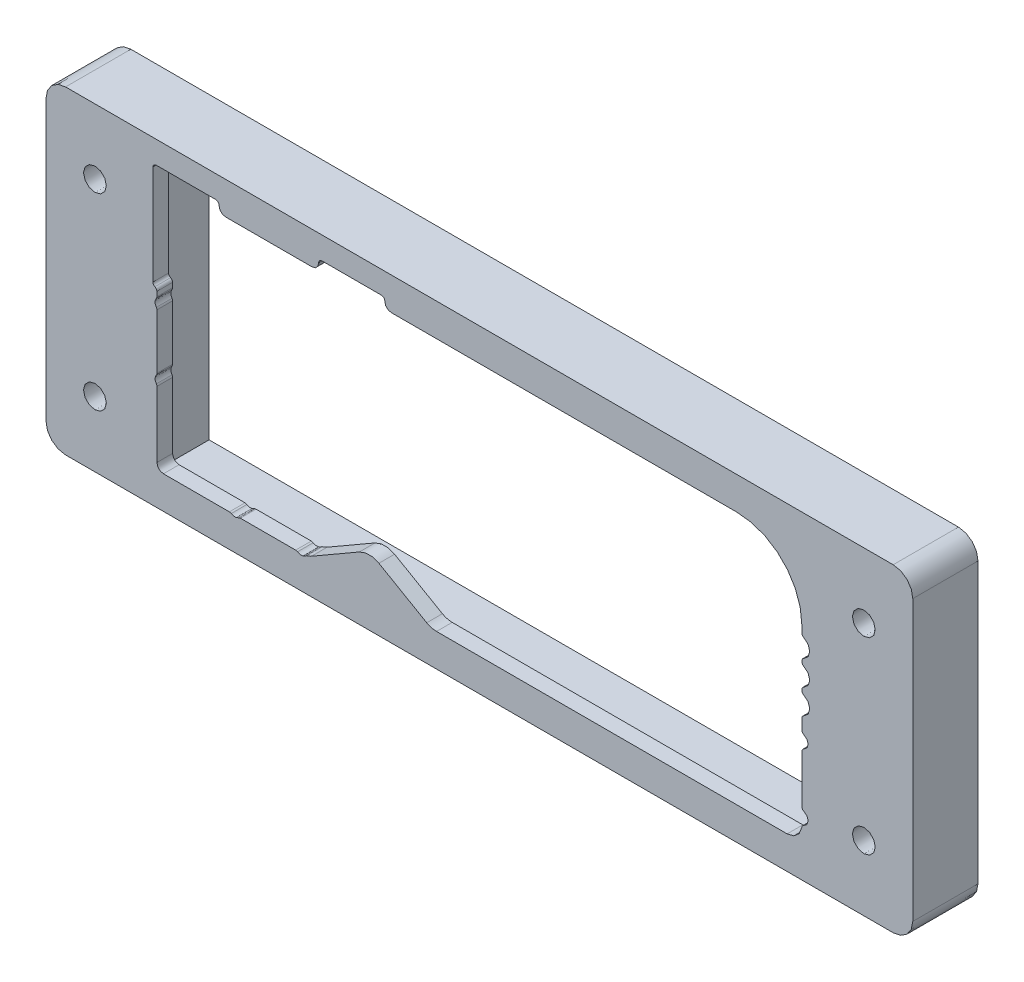
# Autodesk Inventor part: LCD-Halterung
Saved by Autodesk Inventor 2017.3 (Build 213256000, 256)
## iProperties
Part Number: LCD-Halterung
Material: Generisch
Document SubType Name: Modeling
Designer: Nils
Density: 1 g/cm^3
Appearance: Vorgabe
Author: Nils
Autodesk Inventor part; units mm, degrees
ref_plane "YZ Plane" through (0, 0, 0) normal (1, 0, 0) x (0, 1, 0)
ref_plane "XZ Plane" through (0, 0, 0) normal (0, 1, 0) x (-1, 0, 0)
ref_plane "XY Plane" through (0, 0, 0) normal (0, 0, 1) x (1, 0, 0)
sketch "Skizze1" plane through (0, 0, 0) normal (0, 0, 1) x (1, 0, 0)
  circle A0 centre (-4.2343, -14.8275) radius 0.85 projected
  circle A1 centre (35.7657, -14.8275) radius 0.85 projected
  circle A2 centre (-10.8343, -16.0775) radius 0.75 projected
  circle A3 centre (42.3657, -16.0775) radius 0.75 projected
  circle A4 centre (46.4957, 0.0825) radius 0.66 projected
  circle A5 centre (46.4957, 3.8925) radius 0.66 projected
  circle A6 centre (46.4957, 7.7025) radius 0.66 projected
  circle A7 centre (-44.7343, -15.1575) radius 0.5 projected
  circle A8 centre (-29.9543, -17.4975) radius 0.455 projected
  circle A9 centre (-40.1143, -17.4975) radius 0.455 projected
  circle A10 centre (-29.9543, -9.8775) radius 0.455 projected
  circle A11 centre (-40.1143, -9.8775) radius 0.455 projected
  circle A12 centre (-29.9543, 7.5025) radius 0.455 projected
  circle A13 centre (-40.1143, 7.5025) radius 0.455 projected
  circle A14 centre (-29.9543, 15.1225) radius 0.455 projected
  circle A15 centre (-40.1143, 15.1225) radius 0.455 projected
  circle A16 centre (-51.3443, -6.2675) radius 0.455 projected
  circle A17 centre (-51.3443, 3.8925) radius 0.455 projected
  circle A18 centre (-43.7243, -6.2675) radius 0.455 projected
  circle A19 centre (-43.7243, 3.8925) radius 0.455 projected
  circle A20 centre (-26.3443, -6.2675) radius 0.455 projected
  circle A21 centre (-26.3443, 3.8925) radius 0.455 projected
  circle A22 centre (-18.7243, -6.2675) radius 0.455 projected
  circle A23 centre (-18.7243, 3.8925) radius 0.455 projected
  circle A24 centre (-38.8443, -6.2675) radius 0.455 projected
  circle A25 centre (-38.8443, 3.8925) radius 0.455 projected
  circle A26 centre (-31.2243, -6.2675) radius 0.455 projected
  circle A27 centre (-31.2243, 3.8925) radius 0.455 projected
  circle A28 centre (-21.0643, 11.5125) radius 0.455 projected
  circle A29 centre (-23.6043, 11.5125) radius 0.455 projected
  circle A30 centre (-21.0643, 14.0525) radius 0.455 projected
  circle A31 centre (-23.6043, 14.0525) radius 0.455 projected
  circle A32 centre (-21.0643, 16.5925) radius 0.455 projected
  circle A33 centre (-23.6043, 16.5925) radius 0.455 projected
  circle A34 centre (-46.4643, 11.5125) radius 0.455 projected
  circle A35 centre (-49.0043, 11.5125) radius 0.455 projected
  circle A36 centre (-46.4643, 14.0525) radius 0.455 projected
  circle A37 centre (-49.0043, 14.0525) radius 0.455 projected
  circle A38 centre (-46.4643, 16.5925) radius 0.455 projected
  circle A39 centre (-49.0043, 16.5925) radius 0.455 projected
  circle A40 centre (46.7557, -14.9075) radius 0.405 projected
  circle A41 centre (46.7557, -4.7475) radius 0.405 projected
  circle A42 centre (-47.7343, -10.3575) radius 0.4 projected
  circle A43 centre (-50.7343, -15.1575) radius 0.4 projected
  circle A44 centre (16.3957, -17.6275) radius 0.3 projected
  circle A45 centre (17.6757, -17.6275) radius 0.3 projected
  circle A46 centre (15.1257, -17.6275) radius 0.3 projected
  circle A47 centre (25.2857, -17.6275) radius 0.3 projected
  circle A48 centre (26.5657, -17.6275) radius 0.3 projected
  circle A49 centre (27.8357, -17.6275) radius 0.3 projected
  circle A50 centre (29.0957, -17.6275) radius 0.3 projected
  circle A51 centre (30.3657, -17.6275) radius 0.3 projected
  circle A52 centre (32.9057, -17.6275) radius 0.3 projected
  circle A53 centre (13.8557, -17.6275) radius 0.3 projected
  circle A54 centre (12.5957, -17.6275) radius 0.3 projected
  circle A55 centre (11.3157, -17.6275) radius 0.3 projected
  circle A56 centre (10.0457, -17.6275) radius 0.3 projected
  circle A57 centre (8.7757, -17.6275) radius 0.3 projected
  circle A58 centre (7.5057, -17.6275) radius 0.3 projected
  circle A59 centre (6.2457, -17.6275) radius 0.3 projected
  circle A60 centre (4.9657, -17.6275) radius 0.3 projected
  circle A61 centre (-1.3843, -17.6275) radius 0.3 projected
  circle A62 centre (18.9357, -17.6275) radius 0.3 projected
  circle A63 centre (24.0157, -17.6275) radius 0.3 projected
  circle A64 centre (22.7457, -17.6275) radius 0.3 projected
  circle A65 centre (20.2057, -17.6275) radius 0.3 projected
  circle A66 centre (21.4757, -17.6275) radius 0.3 projected
  circle A67 centre (31.6357, -17.6275) radius 0.3 projected
  circle A68 centre (1.1557, -17.6275) radius 0.3 projected
  circle A69 centre (2.4257, -17.6275) radius 0.3 projected
  circle A70 centre (-0.1143, -17.6275) radius 0.3 projected
  circle A71 centre (3.7057, -17.6275) radius 0.3 projected
  circle A72 centre (26.1797, 7.9565) radius 0.175 projected
  circle A73 centre (24.6557, 3.0035) radius 0.175 projected
  circle A74 centre (16.4007, -1.3145) radius 0.175 projected
  circle A75 centre (16.4007, -0.1715) radius 0.175 projected
  circle A76 centre (16.4007, 1.8605) radius 0.175 projected
  circle A77 centre (-9.8883, 7.0675) radius 0.175 projected
  circle A78 centre (17.5437, 8.3375) radius 0.175 projected
  circle A79 centre (17.5437, 9.3535) radius 0.175 projected
  circle A80 centre (17.5437, 10.3695) radius 0.175 projected
  circle A81 centre (26.1797, 8.7185) radius 0.175 projected
  circle A82 centre (-0.1093, -15.1575) radius 0.175 projected
  circle A83 centre (25.4177, -2.3305) radius 0.175 projected
  circle A84 centre (25.4177, 0.0825) radius 0.175 projected
  circle A85 centre (21.9887, 13.4175) radius 0.175 projected
  circle A86 centre (26.1797, 0.0825) radius 0.175 projected
  circle A87 centre (22.7507, 14.0525) radius 0.175 projected
  circle A88 centre (2.0497, -8.2995) radius 0.175 projected
  circle A89 centre (31.5216, 5.0434) radius 0.175 projected
  circle A90 centre (9.0347, 14.1795) radius 0.175 projected
  circle A91 centre (0.7797, 14.4335) radius 0.175 projected
  circle A92 centre (-2.1413, 14.3065) radius 0.175 projected
  circle A93 centre (14.4957, 11.5125) radius 0.175 projected
  circle A94 centre (-6.7133, -8.2995) radius 0.175 projected
  circle A95 centre (4.7167, -5.6325) radius 0.175 projected
  circle A96 centre (4.7167, 4.5275) radius 0.175 projected
  circle A97 centre (27.8307, -6.6485) radius 0.175 projected
  circle A98 centre (16.6547, -10.2045) radius 0.175 projected
  circle A99 centre (1.1607, -14.3955) radius 0.175 projected
  circle A100 centre (40.7847, 8.2105) radius 0.175 projected
  circle A101 centre (18.5597, 16.0845) radius 0.175 projected
  circle A102 centre (4.3357, 13.7985) radius 0.175 projected
  circle A103 centre (30.6247, 6.9405) radius 0.175 projected
  circle A104 centre (28.9737, 5.2895) radius 0.175 projected
  circle A105 centre (10.0507, -11.2205) radius 0.175 projected
  circle A106 centre (20.9727, 11.7665) radius 0.175 projected
  line L0 (48.7857, -20.2375) -> (-54.0643, -20.2375) projected
  line L1 (48.7857, 22.6125) -> (48.7857, -20.2375) projected
  line L2 (-54.0643, 22.6125) -> (48.7857, 22.6125) projected
  line L3 (-54.0643, -20.2375) -> (-54.0643, 22.6125) projected
  line L4 (60.7857, -23.2375) -> (-66.0643, -23.2375)
  line L5 (-69.0643, -20.2375) -> (-69.0643, 22.6125)
  line L6 (-66.0643, 25.6125) -> (60.7857, 25.6125)
  line L7 (63.7857, 22.6125) -> (63.7857, -20.2375)
  arc A107 (60.7857, -23.2375) -> (63.7857, -20.2375) centre (60.7857, -20.2375) ccw
  arc A108 (63.7857, 22.6125) -> (60.7857, 25.6125) centre (60.7857, 22.6125) ccw
  arc A109 (-66.0643, 25.6125) -> (-69.0643, 22.6125) centre (-66.0643, 22.6125) ccw
  arc A110 (-69.0643, -20.2375) -> (-66.0643, -23.2375) centre (-66.0643, -20.2375) ccw
  point P0 (0, 0)
  dimension "d0" = 3
  dimension "d1" = 3
  dimension "d2" = 15
  dimension "d3" = 15
  dimension "d4" = 3
  constraints: 8 end point, 8 point on circle, 8 tangent, 4 centre point, 3 equal radius, 2 parallel, 1 horizontal, 1 perpendicular
  measures "d0" distance between parallel lines of L4 L0
  measures "d1" distance between parallel lines of L6 L2
  measures "d2" distance between parallel lines of L1 L7
  measures "d3" distance between parallel lines of L5 L3
  measures "d4" radius of A107
extrude "Extrusion1" add sketch "Skizze1" along normal blind 10 contours L4 A110 L5 A109 L6 A108 L7 A107
ref_plane "Arbeitsebene1" through (-2.6393, 1.1875, 7.6) normal (0, 0, 1) x (1, 0, 0)
sketch "Skizze2" plane through (-2.6393, 1.1875, 7.6) normal (0, 0, 1) x (1, 0, 0)
  line L0 (-51.425, -21.425) -> (-51.425, 21.425) projected
  line L1 (-51.425, 21.425) -> (51.425, 21.425) projected
  line L2 (51.425, 21.425) -> (51.425, -21.425) projected
  line L3 (51.425, -21.425) -> (-51.425, -21.425) projected
  line L4 (-63.425, -24.425) -> (63.425, -24.425) projected
  arc A0 (63.425, -24.425) -> (66.425, -21.425) centre (63.425, -21.425) ccw projected
  line L5 (66.425, -21.425) -> (66.425, 21.425) projected
  arc A1 (66.425, 21.425) -> (63.425, 24.425) centre (63.425, 21.425) ccw projected
  line L6 (63.425, 24.425) -> (-63.425, 24.425) projected
  arc A2 (-63.425, 24.425) -> (-66.425, 21.425) centre (-63.425, 21.425) ccw projected
  line L7 (-66.425, 21.425) -> (-66.425, -21.425) projected
  arc A3 (-66.425, -21.425) -> (-63.425, -24.425) centre (-63.425, -21.425) ccw projected
  line L8 (-8.0686, -19.0231) -> (-15.3987, -14.791)
  line L9 (-18.3987, -14.791) -> (-25.7288, -19.0231)
  line L10 (47.175, -19.425) -> (-6.5686, -19.425)
  arc A4 (-15.3987, -14.791) -> (-18.3987, -14.791) centre (-16.8987, -17.3891) ccw
  arc A5 (-26.4463, -19.3211) -> (-25.7288, -19.0231) centre (-27.2288, -16.425) ccw
  arc A6 (-8.0686, -19.0231) -> (-6.5686, -19.425) centre (-6.5686, -16.425) ccw
  arc A7 (-49.425, -18.425) -> (-48.425, -19.425) centre (-48.425, -18.425) ccw
  arc A8 (49.425, 9.425) -> (39.425, 19.425) centre (39.425, 9.425) ccw
  arc A9 (47.175, -19.425) -> (49.4027, -17.4913) centre (47.175, -17.175) ccw
  circle A10 centre (-1.595, -16.015) radius 0.85 construction
  circle A11 centre (38.405, -16.015) radius 0.85 construction
  circle A12 centre (-8.195, -17.265) radius 0.75 construction
  circle A13 centre (45.005, -17.265) radius 0.75 construction
  circle A14 centre (49.135, -1.105) radius 0.66 construction
  circle A15 centre (49.135, 2.705) radius 0.66 construction
  circle A16 centre (49.135, 6.515) radius 0.66 construction
  circle A17 centre (-42.095, -16.345) radius 0.5 construction
  circle A18 centre (-27.315, -18.685) radius 0.455 construction
  circle A19 centre (-37.475, -18.685) radius 0.455 construction
  circle A20 centre (-27.315, -11.065) radius 0.455 construction
  circle A21 centre (-37.475, -11.065) radius 0.455 construction
  circle A22 centre (-27.315, 6.315) radius 0.455 construction
  circle A23 centre (-37.475, 6.315) radius 0.455 construction
  circle A24 centre (-27.315, 13.935) radius 0.455 construction
  circle A25 centre (-37.475, 13.935) radius 0.455 construction
  circle A26 centre (-48.705, -7.455) radius 0.455 construction
  circle A27 centre (-48.705, 2.705) radius 0.455 construction
  circle A28 centre (-41.085, -7.455) radius 0.455 construction
  circle A29 centre (-41.085, 2.705) radius 0.455 construction
  circle A30 centre (-23.705, -7.455) radius 0.455 construction
  circle A31 centre (-23.705, 2.705) radius 0.455 construction
  circle A32 centre (-16.085, -7.455) radius 0.455 construction
  circle A33 centre (-16.085, 2.705) radius 0.455 construction
  circle A34 centre (-36.205, -7.455) radius 0.455 construction
  circle A35 centre (-36.205, 2.705) radius 0.455 construction
  circle A36 centre (-28.585, -7.455) radius 0.455 construction
  circle A37 centre (-28.585, 2.705) radius 0.455 construction
  circle A38 centre (-18.425, 10.325) radius 0.455 construction
  circle A39 centre (-20.965, 10.325) radius 0.455 construction
  circle A40 centre (-18.425, 12.865) radius 0.455 construction
  circle A41 centre (-20.965, 12.865) radius 0.455 construction
  circle A42 centre (-18.425, 15.405) radius 0.455 construction
  circle A43 centre (-20.965, 15.405) radius 0.455 construction
  circle A44 centre (-43.825, 10.325) radius 0.455 construction
  circle A45 centre (-46.365, 10.325) radius 0.455 construction
  circle A46 centre (-43.825, 12.865) radius 0.455 construction
  circle A47 centre (-46.365, 12.865) radius 0.455 construction
  circle A48 centre (-43.825, 15.405) radius 0.455 construction
  circle A49 centre (-46.365, 15.405) radius 0.455 construction
  circle A50 centre (49.395, -16.095) radius 0.405 construction
  circle A51 centre (49.395, -5.935) radius 0.405 construction
  circle A52 centre (-45.095, -11.545) radius 0.4 construction
  circle A53 centre (-48.095, -16.345) radius 0.4 construction
  circle A54 centre (19.035, -18.815) radius 0.3 construction
  circle A55 centre (20.315, -18.815) radius 0.3 construction
  circle A56 centre (17.765, -18.815) radius 0.3 construction
  circle A57 centre (27.925, -18.815) radius 0.3 construction
  circle A58 centre (29.205, -18.815) radius 0.3 construction
  circle A59 centre (30.475, -18.815) radius 0.3 construction
  circle A60 centre (31.735, -18.815) radius 0.3 construction
  circle A61 centre (33.005, -18.815) radius 0.3 construction
  circle A62 centre (35.545, -18.815) radius 0.3 construction
  circle A63 centre (16.495, -18.815) radius 0.3 construction
  circle A64 centre (15.235, -18.815) radius 0.3 construction
  circle A65 centre (13.955, -18.815) radius 0.3 construction
  circle A66 centre (12.685, -18.815) radius 0.3 construction
  circle A67 centre (11.415, -18.815) radius 0.3 construction
  circle A68 centre (10.145, -18.815) radius 0.3 construction
  circle A69 centre (8.885, -18.815) radius 0.3 construction
  circle A70 centre (7.605, -18.815) radius 0.3 construction
  circle A71 centre (1.255, -18.815) radius 0.3 construction
  circle A72 centre (21.575, -18.815) radius 0.3 construction
  circle A73 centre (26.655, -18.815) radius 0.3 construction
  circle A74 centre (25.385, -18.815) radius 0.3 construction
  circle A75 centre (22.845, -18.815) radius 0.3 construction
  circle A76 centre (24.115, -18.815) radius 0.3 construction
  circle A77 centre (34.275, -18.815) radius 0.3 construction
  circle A78 centre (3.795, -18.815) radius 0.3 construction
  circle A79 centre (5.065, -18.815) radius 0.3 construction
  circle A80 centre (2.525, -18.815) radius 0.3 construction
  circle A81 centre (6.345, -18.815) radius 0.3 construction
  circle A82 centre (28.819, 6.769) radius 0.175 construction
  circle A83 centre (27.295, 1.816) radius 0.175 construction
  circle A84 centre (19.04, -2.502) radius 0.175 construction
  circle A85 centre (19.04, -1.359) radius 0.175 construction
  circle A86 centre (19.04, 0.673) radius 0.175 construction
  circle A87 centre (-7.249, 5.88) radius 0.175 construction
  circle A88 centre (20.183, 7.15) radius 0.175 construction
  circle A89 centre (20.183, 8.166) radius 0.175 construction
  circle A90 centre (20.183, 9.182) radius 0.175 construction
  circle A91 centre (28.819, 7.531) radius 0.175 construction
  circle A92 centre (2.53, -16.345) radius 0.175 construction
  circle A93 centre (28.057, -3.518) radius 0.175 construction
  circle A94 centre (28.057, -1.105) radius 0.175 construction
  circle A95 centre (24.628, 12.23) radius 0.175 construction
  circle A96 centre (28.819, -1.105) radius 0.175 construction
  circle A97 centre (25.39, 12.865) radius 0.175 construction
  circle A98 centre (4.689, -9.487) radius 0.175 construction
  circle A99 centre (34.1609, 3.8559) radius 0.175 construction
  circle A100 centre (11.674, 12.992) radius 0.175 construction
  circle A101 centre (3.419, 13.246) radius 0.175 construction
  circle A102 centre (0.498, 13.119) radius 0.175 construction
  circle A103 centre (17.135, 10.325) radius 0.175 construction
  circle A104 centre (-4.074, -9.487) radius 0.175 construction
  circle A105 centre (7.356, -6.82) radius 0.175 construction
  circle A106 centre (7.356, 3.34) radius 0.175 construction
  circle A107 centre (30.47, -7.836) radius 0.175 construction
  circle A108 centre (19.294, -11.392) radius 0.175 construction
  circle A109 centre (3.8, -15.583) radius 0.175 construction
  circle A110 centre (43.424, 7.023) radius 0.175 construction
  circle A111 centre (21.199, 14.897) radius 0.175 construction
  circle A112 centre (6.975, 12.611) radius 0.175 construction
  circle A113 centre (33.264, 5.753) radius 0.175 construction
  circle A114 centre (31.613, 4.102) radius 0.175 construction
  circle A115 centre (12.69, -12.408) radius 0.175 construction
  circle A116 centre (23.612, 10.579) radius 0.175 construction
  line L11 (51.425, -21.425) -> (-51.425, -21.425) construction
  line L12 (51.425, 21.425) -> (51.425, -21.425) construction
  line L13 (-51.425, 21.425) -> (51.425, 21.425) construction
  line L14 (-51.425, -21.425) -> (-51.425, 21.425) construction
  line L15 (-40.396, 5.245) -> (-40.396, 20.485) construction
  line L16 (-40.396, 20.485) -> (-49.54, 20.485) construction
  line L17 (-49.54, 20.485) -> (-49.54, 5.245) construction
  line L18 (-49.54, 5.245) -> (-40.396, 5.245) construction
  line L19 (-14.996, 5.245) -> (-14.996, 20.485) construction
  line L20 (-14.996, 20.485) -> (-24.14, 20.485) construction
  line L21 (-24.14, 20.485) -> (-24.14, 5.245) construction
  line L22 (-24.14, 5.245) -> (-14.996, 5.245) construction
  line L23 (-27.995, -20.075) -> (-27.395, -20.075) construction
  line L24 (-27.395, -20.075) -> (-27.395, -18.895) construction
  line L25 (-28.185, -20.305) -> (-28.3918, -20.305) construction
  line L26 (-28.7782, -20.305) -> (-28.3918, -20.305) construction
  line L27 (-28.7782, -20.305) -> (-28.985, -20.305) construction
  line L28 (-28.985, -20.075) -> (-30.725, -20.075) construction
  line L29 (-31.525, -20.075) -> (-30.725, -20.075) construction
  line L30 (-33.065, -20.075) -> (-34.525, -20.075) construction
  line L31 (-35.595, -20.075) -> (-34.595, -20.075) construction
  line L32 (-36.3982, -20.305) -> (-36.0118, -20.305) construction
  line L33 (-37.395, -20.075) -> (-36.795, -20.075) construction
  line L34 (-37.395, -18.895) -> (-37.395, -20.075) construction
  line L35 (-50.095, -6.195) -> (-50.095, -7.375) construction
  line L36 (-50.095, -6.195) -> (-50.095, -5.555) construction
  line L37 (-50.095, -4.175) -> (-50.095, -0.575) construction
  line L38 (-50.095, 2.625) -> (-50.095, 1.445) construction
  line L39 (-50.095, -7.375) -> (-49.495, -7.375) construction
  line L40 (-49.495, 2.625) -> (-50.095, 2.625) construction
  arc A117 (-27.8777, -19.5117) -> (-26.6489, -19.4309) centre (-27.315, -18.685) ccw
  arc A118 (-38.0377, -19.5117) -> (-36.9123, -19.5117) centre (-37.475, -18.685) ccw
  line L41 (-28.159, -19.425) -> (-36.631, -19.425)
  line L42 (-38.319, -19.425) -> (-48.425, -19.425)
  arc A119 (49.7333, -17.036) -> (49.7483, -15.1595) centre (49.395, -16.095) ccw
  arc A120 (49.7483, -6.8705) -> (49.7483, -4.9995) centre (49.395, -5.935) ccw
  arc A121 (49.7275, -2.483) -> (49.7275, 0.273) centre (49.135, -1.105) ccw
  arc A122 (49.7275, 1.327) -> (49.7275, 4.083) centre (49.135, 2.705) ccw
  arc A123 (49.7275, 5.137) -> (49.7275, 7.893) centre (49.135, 6.515) ccw
  line L43 (49.425, -7.3382) -> (49.425, -14.6918)
  line L44 (49.425, -2.9424) -> (49.425, -4.5318)
  line L45 (49.425, 0.8676) -> (49.425, 0.7324)
  line L46 (49.425, 9.425) -> (49.425, 8.3524)
  line L47 (49.425, 4.6776) -> (49.425, 4.5424)
  line L48 (-24.64, 20.425) -> (-24.64, 20.485)
  line L49 (-24.14, 20.985) -> (-14.996, 20.985)
  line L50 (-14.496, 20.485) -> (-14.496, 20.425)
  line L51 (-50.04, 5.2116) -> (-50.04, 20.485)
  line L52 (-49.54, 20.985) -> (-40.396, 20.985)
  line L53 (-39.896, 20.485) -> (-39.896, 20.425)
  line L54 (-38.896, 19.425) -> (-25.64, 19.425)
  line L55 (-13.496, 19.425) -> (39.425, 19.425)
  arc A124 (-49.5183, -6.8732) -> (-49.5183, -8.0368) centre (-48.705, -7.455) ccw
  arc A125 (-49.5183, 3.2868) -> (-49.5183, 2.1232) centre (-48.705, 2.705) ccw
  line L56 (-49.425, 3.5777) -> (-49.425, 4.2884)
  line L57 (-49.425, -18.425) -> (-49.425, -8.3277)
  line L58 (-49.425, -6.5823) -> (-49.425, 1.8323)
  arc A126 (-14.496, 20.425) -> (-13.496, 19.425) centre (-13.496, 20.425) ccw
  arc A127 (-25.64, 19.425) -> (-24.64, 20.425) centre (-25.64, 20.425) ccw
  arc A128 (-39.896, 20.425) -> (-38.896, 19.425) centre (-38.896, 20.425) ccw
  arc A129 (-49.425, 4.2884) -> (-49.7326, 4.7502) centre (-49.9255, 4.2884) ccw
  arc A130 (49.425, 8.3524) -> (49.7275, 7.893) centre (49.925, 8.3524) ccw
  arc A131 (49.7275, 5.137) -> (49.425, 4.6776) centre (49.925, 4.6776) ccw
  arc A132 (49.425, 4.5424) -> (49.7275, 4.083) centre (49.925, 4.5424) ccw
  arc A133 (49.7275, 1.327) -> (49.425, 0.8676) centre (49.925, 0.8676) ccw
  arc A134 (49.425, 0.7324) -> (49.7275, 0.273) centre (49.925, 0.7324) ccw
  arc A135 (49.7275, -2.483) -> (49.425, -2.9424) centre (49.925, -2.9424) ccw
  arc A136 (49.425, -4.5318) -> (49.7483, -4.9995) centre (49.925, -4.5318) ccw
  arc A137 (49.7483, -6.8705) -> (49.425, -7.3382) centre (49.925, -7.3382) ccw
  arc A138 (49.425, -14.6918) -> (49.7483, -15.1595) centre (49.925, -14.6918) ccw
  arc A139 (49.7333, -17.036) -> (49.4027, -17.4913) centre (49.9024, -17.5066) ccw
  arc A140 (-39.896, 20.485) -> (-40.396, 20.985) centre (-40.396, 20.485) ccw
  arc A141 (-49.54, 20.985) -> (-50.04, 20.485) centre (-49.54, 20.485) ccw
  arc A142 (-24.14, 20.985) -> (-24.64, 20.485) centre (-24.14, 20.485) ccw
  arc A143 (-14.496, 20.485) -> (-14.996, 20.985) centre (-14.996, 20.485) ccw
  arc A144 (-50.04, 5.2116) -> (-49.7326, 4.7502) centre (-49.54, 5.2116) ccw
  arc A145 (-49.5183, 3.2868) -> (-49.425, 3.5777) centre (-49.925, 3.5777) ccw
  arc A146 (-49.425, 1.8323) -> (-49.5183, 2.1232) centre (-49.925, 1.8323) ccw
  arc A147 (-49.5183, -6.8732) -> (-49.425, -6.5823) centre (-49.925, -6.5823) ccw
  arc A148 (-49.425, -8.3277) -> (-49.5183, -8.0368) centre (-49.925, -8.3277) ccw
  arc A149 (-38.0377, -19.5117) -> (-38.319, -19.425) centre (-38.319, -19.925) ccw
  arc A150 (-36.631, -19.425) -> (-36.9123, -19.5117) centre (-36.631, -19.925) ccw
  arc A151 (-27.8777, -19.5117) -> (-28.159, -19.425) centre (-28.159, -19.925) ccw
  arc A152 (-26.4463, -19.3211) -> (-26.6489, -19.4309) centre (-26.3159, -19.8038) ccw
  point P0 (2.6393, -1.1875)
  point P1 (-49.425, -19.425)
  point P2 (-7.3724, -19.425)
  point P3 (-16.8987, -13.925)
  point P4 (-26.425, -19.425)
  point P5 (-49.425, 4.745)
  point P6 (-27.9876, -19.425)
  point P7 (-38.1476, -19.425)
  point P8 (-36.8024, -19.425)
  point P9 (49.425, -15.0955)
  point P10 (49.425, -17.0945)
  point P11 (49.425, -6.9345)
  point P12 (49.425, -4.9355)
  point P13 (49.425, -2.5767)
  point P14 (49.425, 0.3667)
  point P15 (49.425, 1.2333)
  point P16 (49.425, 4.1767)
  point P17 (49.425, 5.0433)
  point P18 (49.425, 7.9867)
  point P19 (-14.496, 19.425)
  point P20 (-24.64, 20.985)
  point P21 (-14.496, 20.985)
  point P22 (-50.04, 20.985)
  point P23 (-50.04, 4.745)
  point P24 (-39.896, 20.985)
  point P25 (-24.64, 19.425)
  point P26 (-39.896, 19.425)
  point P27 (-49.425, 2.011)
  point P28 (-49.425, 3.399)
  point P29 (-49.425, -8.149)
  point P30 (-49.425, -6.761)
  dimension "d11" = 120
  dimension "d13" = 23
  dimension "d14" = 2
  dimension "d16" = 5.5
  dimension "d17" = 3
  dimension "d18" = 3
  dimension "d19" = 1
  dimension "d20" = 2
  dimension "d21" = 2
  dimension "d22" = 2
  dimension "d23" = 2
  dimension "d24" = 3
  dimension "d25" = 3
  dimension "d26" = 3
  dimension "d27" = 0.5
  dimension "d28" = 0.5
  dimension "d29" = 0.5
  dimension "d30" = 0.5
  dimension "d31" = 0.5
  dimension "d33" = 2
  dimension "d34" = 2
  dimension "d37" = 2
  dimension "d38" = 2
  dimension "d39" = 10
  dimension "d40" = 2.25
  dimension "d52" = 1
  dimension "d54" = 0.5
  dimension "d55" = 0.5
  dimension "d56" = 0.5
  constraints: 101 point on circle, 77 tangent, 42 centre point, 42 end point, 38 point on line, 23 equal radius, 23 parallel, 9 coincident, 9 perpendicular, 3 horizontal, 1 equal length, 1 other
  measures "d11" angle of L9 L8
  measures "d13" distance of point (-49.425, -19.425) point (-26.425, -19.425)
  measures "d14" distance between parallel lines of L3 L10
  measures "d16" vertical distance of point (-7.372, -19.425) point (-16.899, -13.925)
  measures "d17" radius of A4
  measures "d18" radius of A6
  measures "d19" radius of A7
  measures "d20" diameter of A117
  measures "d21" diameter of A118
  measures "d22" diameter of A119
  measures "d23" diameter of A120
  measures "d24" diameter of A121
  measures "d25" diameter of A122
  measures "d26" diameter of A123
  measures "d27" distance between parallel lines of L20 L49
  measures "d28" distance between parallel lines of L19 L50
  measures "d29" distance between parallel lines of L48 L21
  measures "d30" distance between parallel lines of L15 L53
  measures "d31" distance between parallel lines of L51 L17
  measures "d33" diameter of A124
  measures "d34" diameter of A125
  measures "d37" distance between parallel lines of L2 L46
  measures "d38" distance between parallel lines of L13 L55
  measures "d39" radius of A8
  measures "d40" radius of A9
  measures "d52" radius of A126
  measures "d54" radius of A130
  measures "d55" radius of A140
  measures "d56" radius of A145
extrude "Extrusion2" add sketch "Skizze2" along normal up to surface (2.4 mm away) contours L0 L1 L2 L3
sketch "Skizze3" plane through (0, 0, 10) normal (0, 0, 1) x (1, 0, 0)
  arc A0 (-29.0856, -18.1337) -> (-28.3681, -17.8356) centre (-29.8681, -15.2375) ccw construction
  arc A1 (-30.517, -18.3242) -> (-29.2882, -18.2434) centre (-29.9543, -17.4975) ccw construction
  line L0 (-39.2703, -18.2375) -> (-30.7983, -18.2375) construction
  arc A2 (-40.677, -18.3242) -> (-39.5516, -18.3242) centre (-40.1143, -17.4975) ccw construction
  line L1 (-51.0643, -18.2375) -> (-40.9583, -18.2375) construction
  arc A3 (-52.0643, -17.2375) -> (-51.0643, -18.2375) centre (-51.0643, -17.2375) ccw construction
  line L2 (-52.0643, -7.1403) -> (-52.0643, -17.2375) construction
  arc A4 (-52.1576, -5.6857) -> (-52.1576, -6.8493) centre (-51.3443, -6.2675) ccw construction
  line L3 (-52.0643, 3.0197) -> (-52.0643, -5.3948) construction
  arc A5 (-52.1576, 4.4743) -> (-52.1576, 3.3107) centre (-51.3443, 3.8925) ccw construction
  line L4 (-52.0643, 5.4759) -> (-52.0643, 4.7652) construction
  line L5 (-52.6793, 21.6725) -> (-52.6793, 6.3991) construction
  line L6 (-43.0353, 22.1725) -> (-52.1793, 22.1725) construction
  line L7 (-42.5353, 21.6125) -> (-42.5353, 21.6725) construction
  line L8 (-28.2793, 20.6125) -> (-41.5353, 20.6125) construction
  line L9 (-27.2793, 21.6725) -> (-27.2793, 21.6125) construction
  line L10 (-17.6353, 22.1725) -> (-26.7793, 22.1725) construction
  line L11 (-17.1353, 21.6125) -> (-17.1353, 21.6725) construction
  line L12 (36.7857, 20.6125) -> (-16.1353, 20.6125) construction
  arc A6 (46.7857, 10.6125) -> (36.7857, 20.6125) centre (36.7857, 10.6125) ccw construction
  line L13 (46.7857, 9.5398) -> (46.7857, 10.6125) construction
  arc A7 (47.0882, 6.3245) -> (47.0882, 9.0805) centre (46.4957, 7.7025) ccw construction
  line L14 (46.7857, 5.7298) -> (46.7857, 5.8651) construction
  arc A8 (47.0882, 2.5145) -> (47.0882, 5.2705) centre (46.4957, 3.8925) ccw construction
  line L15 (46.7857, 1.9198) -> (46.7857, 2.0551) construction
  arc A9 (47.0882, -1.2955) -> (47.0882, 1.4605) centre (46.4957, 0.0825) ccw construction
  line L16 (46.7857, -3.3443) -> (46.7857, -1.7549) construction
  arc A10 (47.109, -5.683) -> (47.109, -3.812) centre (46.7557, -4.7475) ccw construction
  line L17 (46.7857, -13.5043) -> (46.7857, -6.1508) construction
  arc A11 (47.094, -15.8486) -> (47.109, -13.972) centre (46.7557, -14.9075) ccw construction
  arc A12 (44.5357, -18.2375) -> (46.7634, -16.3039) centre (44.5357, -15.9875) ccw construction
  line L18 (-9.2079, -18.2375) -> (44.5357, -18.2375) construction
  arc A13 (-10.7079, -17.8356) -> (-9.2079, -18.2375) centre (-9.2079, -15.2375) ccw construction
  line L19 (-18.038, -13.6035) -> (-10.7079, -17.8356) construction
  arc A14 (-18.038, -13.6035) -> (-21.038, -13.6035) centre (-19.538, -16.2016) ccw construction
  line L20 (-28.3681, -17.8356) -> (-21.038, -13.6035) construction
  line L21 (-66.0643, -23.2375) -> (60.7857, -23.2375) construction
  arc A15 (60.7857, -23.2375) -> (63.7857, -20.2375) centre (60.7857, -20.2375) ccw construction
  line L22 (63.7857, -20.2375) -> (63.7857, 22.6125) construction
  arc A16 (63.7857, 22.6125) -> (60.7857, 25.6125) centre (60.7857, 22.6125) ccw construction
  line L23 (60.7857, 25.6125) -> (-66.0643, 25.6125) construction
  arc A17 (-66.0643, 25.6125) -> (-69.0643, 22.6125) centre (-66.0643, 22.6125) ccw construction
  line L24 (-69.0643, 22.6125) -> (-69.0643, -20.2375) construction
  arc A18 (-69.0643, -20.2375) -> (-66.0643, -23.2375) centre (-66.0643, -20.2375) ccw construction
  arc A19 (-52.0643, 5.4759) -> (-52.3719, 5.9377) centre (-52.5648, 5.4759) ccw projected
  arc A20 (-42.5353, 21.6125) -> (-41.5353, 20.6125) centre (-41.5353, 21.6125) ccw projected
  arc A21 (-28.2793, 20.6125) -> (-27.2793, 21.6125) centre (-28.2793, 21.6125) ccw projected
  arc A22 (-17.1353, 21.6125) -> (-16.1353, 20.6125) centre (-16.1353, 21.6125) ccw projected
  arc A23 (-29.0856, -18.1337) -> (-29.2882, -18.2434) centre (-28.9552, -18.6164) ccw projected
  arc A24 (-30.517, -18.3242) -> (-30.7983, -18.2375) centre (-30.7983, -18.7375) ccw projected
  arc A25 (-39.2703, -18.2375) -> (-39.5516, -18.3242) centre (-39.2703, -18.7375) ccw projected
  arc A26 (-40.677, -18.3242) -> (-40.9583, -18.2375) centre (-40.9583, -18.7375) ccw projected
  arc A27 (-52.0643, -7.1403) -> (-52.1576, -6.8493) centre (-52.5643, -7.1403) ccw projected
  arc A28 (-52.1576, -5.6857) -> (-52.0643, -5.3948) centre (-52.5643, -5.3948) ccw projected
  arc A29 (-52.0643, 3.0197) -> (-52.1576, 3.3107) centre (-52.5643, 3.0197) ccw projected
  arc A30 (-52.1576, 4.4743) -> (-52.0643, 4.7652) centre (-52.5643, 4.7652) ccw projected
  arc A31 (-52.6793, 6.3991) -> (-52.3719, 5.9377) centre (-52.1793, 6.3991) ccw projected
  arc A32 (-52.1793, 22.1725) -> (-52.6793, 21.6725) centre (-52.1793, 21.6725) ccw projected
  arc A33 (-42.5353, 21.6725) -> (-43.0353, 22.1725) centre (-43.0353, 21.6725) ccw projected
  arc A34 (-26.7793, 22.1725) -> (-27.2793, 21.6725) centre (-26.7793, 21.6725) ccw projected
  arc A35 (-17.1353, 21.6725) -> (-17.6353, 22.1725) centre (-17.6353, 21.6725) ccw projected
  arc A36 (46.7857, 9.5398) -> (47.0882, 9.0805) centre (47.2857, 9.5398) ccw projected
  arc A37 (47.0882, 6.3245) -> (46.7857, 5.8651) centre (47.2857, 5.8651) ccw projected
  arc A38 (46.7857, 5.7298) -> (47.0882, 5.2705) centre (47.2857, 5.7298) ccw projected
  arc A39 (47.0882, 2.5145) -> (46.7857, 2.0551) centre (47.2857, 2.0551) ccw projected
  arc A40 (46.7857, 1.9198) -> (47.0882, 1.4605) centre (47.2857, 1.9198) ccw projected
  arc A41 (47.0882, -1.2955) -> (46.7857, -1.7549) centre (47.2857, -1.7549) ccw projected
  arc A42 (46.7857, -3.3443) -> (47.109, -3.812) centre (47.2857, -3.3443) ccw projected
  arc A43 (47.109, -5.683) -> (46.7857, -6.1508) centre (47.2857, -6.1508) ccw projected
  arc A44 (46.7857, -13.5043) -> (47.109, -13.972) centre (47.2857, -13.5043) ccw projected
  arc A45 (47.094, -15.8486) -> (46.7634, -16.3039) centre (47.2631, -16.3191) ccw projected
  point P0 (0, 0)
  point P1 (56.2857, -13.2375)
  point P2 (56.2857, 15.6125)
  point P3 (-61.5643, -13.2375)
  point P4 (-61.5643, 15.6125)
  dimension "d41" = 7.5
  dimension "d42" = 7.5
  dimension "d43" = 10
  dimension "d44" = 10
  constraints: 2 horizontal alignment, 2 vertical alignment
  measures "d41" distance from line of L22 point (56.286, -13.238)
  measures "d42" distance from line of L24 point (-61.564, -13.238)
  measures "d43" distance from line of L21 point (56.286, -13.238)
  measures "d44" distance from line of L23 point (56.286, 15.612)
hole "Bohrung1" at (56.2857, -13.2375, 10) at (56.2857, 15.6125, 10) at (-61.5643, -13.2375, 10) at (-61.5643, 15.6125, 10) direction (0, 0, -1) diameter 3.5 end through all
equation "\"d1\" = d0"
equation "\"d3\" = d2"
equation "\"d14\" = d7"
equation "\"d28\" = d27"
equation "\"d29\" = d27"
equation "\"d30\" = d27"
equation "\"d31\" = d27"
equation "\"d42\" = d41"
equation "\"d44\" = d43"
equation "\"d8\" = d7"
equation "\"d9\" = d7"
equation "\"d10\" = d7"
equation "\"d15\" = d7"
equation "\"d7\" = 2"
